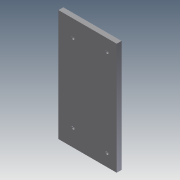
# Autodesk Inventor part: bottombase
Saved by Autodesk Inventor 2011 (Build 150239000, 239)
## iProperties
Created: 2011-12-11
Part Number: bottombase
Document SubType Name: Modeling
Designer: Matthew
Density: 1 g/cm^3
Author: Matthew
Autodesk Inventor part; units mm, degrees
ref_plane "YZ Plane" through (0, 0, 0) normal (1, 0, 0) x (0, 1, 0)
ref_plane "XZ Plane" through (0, 0, 0) normal (0, 1, 0) x (-1, 0, 0)
ref_plane "XY Plane" through (0, 0, 0) normal (0, 0, 1) x (1, 0, 0)
sketch "Sketch1" plane through (0, 0, 0) normal (0, 0, 1) x (1, 0, 0)
  line L0 (-27.8098, 14.1571) -> (47.1902, 14.1571)
  line L1 (47.1902, 14.1571) -> (47.1902, -138.2429)
  line L2 (47.1902, -138.2429) -> (-27.8098, -138.2429)
  line L3 (-27.8098, -138.2429) -> (-27.8098, 14.1571)
  point P0 (0, 0)
  dimension "d0" = 75
  dimension "d1" = 152.4
  constraints: 8 end point, 2 parallel, 1 horizontal, 1 perpendicular
  measures "d0" distance of L1.end L2.end
  measures "d1" distance of L0.end L1.end
extrude "Extrusion1" add sketch "Sketch1" along normal blind 6.35
sketch "Sketch2" plane through (0, 0, 6.35) normal (0, 0, 1) x (1, 0, 0)
  line L0 (47.1902, 14.1571) -> (47.1902, -138.2429) projected
  line L1 (-27.8098, -138.2429) -> (47.1902, -138.2429)
  line L2 (47.1902, -138.2429) -> (47.1902, -125.5429)
  line L3 (47.1902, -125.5429) -> (-27.8098, -125.5429)
  line L4 (-27.8098, -125.5429) -> (-27.8098, -138.2429)
  point P0 (0, 0)
  dimension "d4" = 12.7
  constraints: 8 end point, 2 parallel, 1 horizontal, 1 perpendicular, 1 point on line
  measures "d4" distance of L2.end L1.end
extrude "Extrusion2" cut sketch "Sketch2" against normal blind 25.4
sketch "Sketch3" plane through (0, 0, 6.35) normal (0, 0, 1) x (1, 0, 0)
  line L0 (47.1902, -125.5429) -> (34.4902, -125.5429)
  line L1 (34.4902, -125.5429) -> (34.4902, -112.8429)
  line L2 (34.4902, -112.8429) -> (47.1902, -112.8429)
  line L3 (47.1902, -112.8429) -> (47.1902, -125.5429)
  line L4 (-27.8098, -125.5429) -> (-8.7598, -125.5429)
  line L5 (-8.7598, -125.5429) -> (-8.7598, -106.4929)
  line L6 (-8.7598, -106.4929) -> (-27.8098, -106.4929)
  line L7 (-27.8098, -106.4929) -> (-27.8098, -125.5429)
  line L8 (-27.8098, 14.1571) -> (-8.7598, 14.1571)
  line L9 (-8.7598, 14.1571) -> (-8.7598, -4.8592)
  line L10 (-8.7598, -4.8592) -> (-27.8098, -4.8592)
  line L11 (-27.8098, -4.8592) -> (-27.8098, 14.1571)
  line L12 (47.1902, 14.1571) -> (34.4902, 14.1571)
  line L13 (34.4902, 14.1571) -> (34.4902, 1.4571)
  line L14 (34.4902, 1.4571) -> (47.1902, 1.4571)
  line L15 (47.1902, 1.4571) -> (47.1902, 14.1571)
  circle A0 centre (-8.7598, -106.4929) radius 1.9812
  circle A1 centre (-8.7598, -4.8592) radius 1.9812
  circle A2 centre (34.4902, 1.4571) radius 1.9812
  circle A3 centre (34.4902, -112.8429) radius 1.9812
  point P0 (0, 0)
  dimension "d7" = 12.7
  dimension "d8" = 12.7
  dimension "d9" = 19.05
  dimension "d10" = 19.05
  dimension "d11" = 19.05
  dimension "d12" = 12.7
  dimension "d13" = 12.7
  dimension "d14" = 3.9624
  dimension "d15" = 3.9624
  constraints: 32 end point, 8 parallel, 4 centre point, 4 coincident, 4 horizontal, 4 perpendicular
  measures "d7" distance of L1.end L2.end
  measures "d8" distance of L0.end L1.end
  measures "d9" distance of L6.end L5.end
  measures "d10" distance of L5.end L4.end
  measures "d11" distance of L9.end L10.end
  measures "d12" distance of L14.end L13.end
  measures "d13" distance of L13.end L12.end
  measures "d14" diameter of A0
  measures "d15" diameter of A2
extrude "Extrusion3" cut sketch "Sketch3" against normal blind 25.4 contours A3 L2 L1 | L1 L2 A3 | A0 L6 L5 | L5 L6 A0 | A1 L10 L9 | L9 L10 A1 | A2 L14 L13 | L13 L14 A2
sketch "Sketch4" plane through (0, 0, 6.35) normal (0, 0, 1) x (1, 0, 0)
  circle A0 centre (34.4902, -112.8429) radius 1.9812 projected
  circle A1 centre (34.4902, 1.4571) radius 1.9812 projected
  point P0 (0, 0)
extrude "Extrusion4" add sketch "Sketch4" against normal blind 6.35
sketch "Sketch5" plane through (-27.8098, 14.1571, 0) normal (-1, 0, 0) x (0, 0, 1)
  line L0 (0, -139.7) -> (0, 0) projected
  line L1 (6.35, 0) -> (0, 0)
  line L2 (0, 0) -> (0, -6.9273)
  line L3 (0, -6.9273) -> (6.35, -6.9273)
  line L4 (6.35, -6.9273) -> (6.35, 0)
  point P0 (0, -14.1571)
  constraints: 8 end point, 2 parallel, 1 horizontal, 1 perpendicular, 1 point on line
extrude "Extrusion5" add sketch "Sketch5" against normal blind 76.2
sketch "Sketch6" plane through (48.3902, 14.1571, 0) normal (1, 0, 0) x (0, 0, -1)
  line L0 (0, 0) -> (0, -6.9273) projected
  line L1 (-6.35, 0) -> (0, 0) projected
  line L2 (-6.35, -6.9273) -> (-6.35, 0) projected
  line L3 (0, -6.9273) -> (-6.35, -6.9273) projected
  line L4 (-6.35, 0) -> (0, 0)
  line L5 (0, 0) -> (0, -139.7)
  line L6 (0, -139.7) -> (-6.35, -139.7)
  line L7 (-6.35, -139.7) -> (-6.35, 0)
  point P0 (0, -14.1571)
  dimension "d22" = 139.7
  constraints: 8 end point, 2 parallel, 1 horizontal, 1 perpendicular
  measures "d22" distance of L4.end L5.end
extrude "Extrusion6" add sketch "Sketch6" against normal blind 2.54 contours L5 L6 L7 L3
sketch "Sketch7" plane through (0, 0, 6.35) normal (0, 0, 1) x (1, 0, 0)
  line L0 (48.3902, -125.5429) -> (35.6902, -125.5429)
  line L1 (35.6902, -125.5429) -> (35.6902, -112.8429)
  line L2 (35.6902, -112.8429) -> (48.3902, -112.8429)
  line L3 (48.3902, -112.8429) -> (48.3902, -125.5429)
  line L4 (48.3902, 14.1571) -> (35.6902, 14.1571)
  line L5 (35.6902, 14.1571) -> (35.6902, 1.4571)
  line L6 (35.6902, 1.4571) -> (48.3902, 1.4571)
  line L7 (48.3902, 1.4571) -> (48.3902, 14.1571)
  circle A0 centre (35.6902, -112.8429) radius 1.9812
  circle A1 centre (35.6902, 1.4571) radius 1.9812
  point P0 (0, 0)
  dimension "d25" = 12.7
  dimension "d26" = 12.7
  dimension "d27" = 12.7
  dimension "d28" = 12.7
  dimension "d29" = 3.9624
  dimension "d30" = 3.9624
  constraints: 16 end point, 4 parallel, 2 centre point, 2 coincident, 2 horizontal, 2 perpendicular
  measures "d25" distance of L1.end L2.end
  measures "d26" distance of L0.end L1.end
  measures "d27" distance of L6.end L5.end
  measures "d28" distance of L5.end L4.end
  measures "d29" diameter of A0
  measures "d30" diameter of A1
extrude "Extrusion7" cut sketch "Sketch7" against normal blind 25.4 contours A0 L2 L1 | L1 L2 A0 | A1 L6 L5 | L5 L6 A1
sketch "Sketch8" plane through (-27.8098, -125.5429, 0) normal (0, -1, 0) x (1, 0, 0)
  line L0 (0, 6.35) -> (76.2, 6.35) projected
  line L1 (0, 0) -> (0, 6.35) projected
  line L2 (76.2, 0) -> (0, 0) projected
  line L3 (76.2, 6.35) -> (76.2, 0) projected
  point P0 (27.8098, 0)
extrude "Extrusion8" add sketch "Sketch8" along normal blind 3.175
sketch "Sketch9" plane through (-27.8098, 14.1571, 6.35) normal (0, 1, 0) x (1, 0, 0)
  line L0 (0, 0) -> (76.2, 0) projected
  line L1 (76.2, 0) -> (76.2, 6.35) projected
  line L2 (0, 6.35) -> (76.2, 6.35) projected
  line L3 (0, 6.35) -> (0, 0) projected
  point P0 (27.8098, 6.35)
extrude "Extrusion9" add sketch "Sketch9" along normal blind 3.175
body "Solid1"
